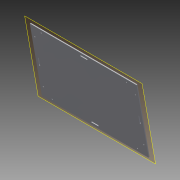
# Autodesk Inventor part: Panel_bottom
Saved by Autodesk Inventor 2013 (Build 170138000, 138)
## iProperties
Created: 2013-02-02
Part Number: Panel_bottom
Material: Aluminum 6061
Document SubType Name: Modeling
Designer: xylzlyx
Density: 1 g/cm^3
Author: xylzlyx
Autodesk Inventor part; units mm, degrees
ref_plane "YZ Plane" through (0, 0, 0) normal (1, 0, 0) x (0, 1, 0)
ref_plane "XZ Plane" through (0, 0, 0) normal (0, 1, 0) x (-1, 0, 0)
ref_plane "XY Plane" through (0, 0, 0) normal (0, 0, 1) x (1, 0, 0)
ref_plane "10DegOffset" through (-190.5, -127, 0) normal (0, -0.1736482, 0.9848078) x (1, 0, 0)
sketch "BottomDimensions" plane through (-190.5, -127, 0) normal (0, -0.1736482, 0.9848078) x (1, 0, 0)
  line L0 (380, 250.1412) -> (1, 250.1412) construction
  line L1 (0, 249.1564) -> (0, 0.9848) construction
  line L2 (381, 0.9848) -> (381, 249.1564) construction
  line L3 (1, 0) -> (380, 0) construction
  line L4 (0, 250.1412) -> (381, 250.1412)
  line L5 (381, 250.1412) -> (381, 0)
  line L6 (381, 0) -> (0, 0)
  line L7 (0, 0) -> (0, 250.1412)
  point P0 (190.5, 125.0706)
  constraints: 8 end point, 2 horizontal alignment, 2 parallel, 2 vertical alignment, 1 horizontal, 1 perpendicular
extrude "Panel" add sketch "BottomDimensions" along normal blind 3.175
fillet "CornerFillets" radius 1 4 edges at (-190.5, 119.0653, 44.9999) (190.5, 119.0653, 44.9999) (190.5, -127.2757, 1.5634) (-190.5, -127.2757, 1.5634)
sketch "ScrewHoleSketch" plane through (-190.5, -127.5513, 3.1268) normal (0, -0.1736482, 0.9848078) x (1, 0, 0)
  line L0 (9.525, 40.9987) -> (12.7, 40.9987) projected
  line L1 (12.7, 37.2014) -> (9.525, 37.2014) projected
  line L2 (12.7, 209.1425) -> (9.525, 209.1425) projected
  line L3 (9.525, 212.9398) -> (12.7, 212.9398) projected
  line L4 (39.9986, 240.6162) -> (39.9986, 237.4412) projected
  line L5 (36.2013, 237.4412) -> (36.2013, 240.6162) projected
  line L6 (188.6014, 237.4412) -> (188.6014, 240.6162) projected
  line L7 (192.3987, 240.6162) -> (192.3987, 237.4412) projected
  line L8 (344.7986, 240.6162) -> (344.7986, 237.4412) projected
  line L9 (341.0013, 237.4412) -> (341.0013, 240.6162) projected
  line L10 (371.475, 209.1425) -> (368.3, 209.1425) projected
  line L11 (368.3, 212.9398) -> (371.475, 212.9398) projected
  line L12 (368.3, 40.9986) -> (371.475, 40.9986) projected
  line L13 (371.475, 37.2013) -> (368.3, 37.2013) projected
  line L14 (341.0014, 9.525) -> (341.0014, 12.7) projected
  line L15 (344.7987, 12.7) -> (344.7987, 9.525) projected
  line L16 (192.3987, 12.7) -> (192.3987, 9.525) projected
  line L17 (188.6014, 9.525) -> (188.6014, 12.7) projected
  line L18 (36.2013, 9.525) -> (36.2013, 12.7) projected
  line L19 (39.9986, 12.7) -> (39.9986, 9.525) projected
  line L20 (9.525, 212.9398) -> (9.525, 209.1425) construction
  line L21 (39.9986, 240.6162) -> (36.2013, 240.6162) construction
  line L22 (344.7986, 240.6162) -> (341.0013, 240.6162) construction
  line L23 (371.475, 209.1425) -> (371.475, 212.9398) construction
  line L24 (368.3, 40.9986) -> (368.3, 37.2013) construction
  line L25 (344.7987, 12.7) -> (341.0014, 12.7) construction
  line L26 (36.2013, 9.525) -> (39.9986, 9.525) construction
  line L27 (12.7, 37.2014) -> (12.7, 40.9987) construction
  point P0 (190.5, 125.0706)
  point P1 (11.1125, 211.0412)
  point P2 (38.1, 239.0287)
  point P3 (342.9, 239.0287)
  point P4 (369.8875, 211.0412)
  point P5 (369.8875, 39.1)
  point P6 (342.9, 11.1125)
  point P7 (36.2013, 239.0287)
  point P8 (9.525, 211.0412)
  point P9 (38.1, 240.6162)
  point P10 (11.1125, 212.9398)
  point P11 (344.7986, 239.0287)
  point P12 (342.9, 240.6162)
  point P13 (369.8875, 212.9398)
  point P14 (371.475, 211.0412)
  point P15 (368.3, 39.1)
  point P16 (341.0014, 11.1125)
  point P17 (369.8875, 40.9986)
  point P18 (342.9, 12.7)
  point P19 (11.1125, 39.1)
  point P20 (38.1, 11.1125)
  point P21 (38.1, 9.525)
  point P22 (11.1125, 37.2014)
  point P23 (12.7, 39.1)
  point P24 (36.2013, 11.1125)
  constraints: 16 end point, 16 midpoint, 8 horizontal alignment, 8 vertical alignment, 2 parallel
hole "ScrewHoles" at (-179.3875, 80.2836, 39.7737) at (-152.4, 107.846, 44.6337) at (152.4, 107.846, 44.6337) at (179.3875, 80.2836, 39.7737) at (179.3875, -89.0453, 9.9164) at (152.4, -116.6077, 5.0564) at (-179.3875, -89.0453, 9.9164) at (-152.4, -116.6077, 5.0564) direction (0, 0.1736482, -0.9848078) diameter 3.7973 end through all
sketch "TabSlotSketch" plane through (-190.5, -127.5513, 3.1268) normal (0, -0.1736482, 0.9848078) x (1, 0, 0)
  circle A0 centre (38.1, 11.1125) radius 1.8986 projected
  circle A1 centre (342.9, 11.1125) radius 1.8986 projected
  circle A2 centre (369.8875, 211.0412) radius 1.8986 projected
  circle A3 centre (38.1, 239.0287) radius 1.8986 projected
  circle A4 centre (342.9, 239.0287) radius 1.8986 projected
  circle A5 centre (369.8875, 39.1) radius 1.8986 projected
  line L0 (12.7, 208.6425) -> (12.7, 41.4986) construction
  line L1 (9.525, 41.4986) -> (9.525, 208.6425) construction
  line L2 (9.525, 213.4398) -> (9.525, 236.4412) construction
  line L3 (12.7, 236.4412) -> (12.7, 213.4398) construction
  line L4 (35.7013, 237.4412) -> (1, 237.4412) construction
  line L5 (1, 240.6162) -> (35.7013, 240.6162) construction
  line L6 (9.525, 13.7) -> (9.525, 36.7013) construction
  line L7 (12.7, 36.7013) -> (12.7, 13.7) construction
  line L8 (1, 12.7) -> (35.7013, 12.7) construction
  line L9 (1, 9.525) -> (35.7013, 9.525) construction
  line L10 (345.2987, 9.525) -> (380, 9.525) construction
  line L11 (345.2987, 12.7) -> (380, 12.7) construction
  line L12 (368.3, 13.7) -> (368.3, 36.7013) construction
  line L13 (371.475, 36.7013) -> (371.475, 13.7) construction
  line L14 (371.475, 208.6425) -> (371.475, 41.4986) construction
  line L15 (368.3, 41.4986) -> (368.3, 208.6425) construction
  line L16 (368.3, 213.4398) -> (368.3, 236.4412) construction
  line L17 (371.475, 236.4412) -> (371.475, 213.4398) construction
  line L18 (380, 237.4412) -> (345.2986, 237.4412) construction
  line L19 (345.2986, 240.6162) -> (380, 240.6162) construction
  line L20 (340.5013, 237.4412) -> (40.4986, 237.4412) construction
  line L21 (40.4986, 240.6162) -> (340.5013, 240.6162) construction
  line L22 (40.4986, 9.525) -> (340.5014, 9.525) construction
  line L23 (40.4986, 12.7) -> (340.5014, 12.7) construction
  line L24 (13.0175, 138.4056) -> (9.2075, 138.4056)
  line L25 (9.2075, 138.4056) -> (9.2075, 111.7356)
  line L26 (9.2075, 111.7356) -> (13.0175, 111.7356)
  line L27 (13.0175, 111.7356) -> (13.0175, 138.4056)
  line L28 (371.7925, 111.7356) -> (367.9825, 111.7356)
  line L29 (367.9825, 111.7356) -> (367.9825, 138.4056)
  line L30 (367.9825, 138.4056) -> (371.7925, 138.4056)
  line L31 (371.7925, 138.4056) -> (371.7925, 111.7356)
  line L32 (9.525, 236.4412) -> (12.7, 236.4412) construction
  line L33 (9.525, 13.7) -> (12.7, 13.7) construction
  line L34 (11.1125, 13.7) -> (11.1125, 236.4412) construction
  line L35 (9.2075, 125.0706) -> (13.0175, 125.0706) construction
  line L36 (11.1125, 138.4056) -> (11.1125, 111.7356) construction
  line L37 (369.8875, 211.0412) -> (369.8875, 39.1) construction
  line L38 (177.165, 240.9337) -> (203.835, 240.9337)
  line L39 (203.835, 240.9337) -> (203.835, 237.1237)
  line L40 (203.835, 237.1237) -> (177.165, 237.1237)
  line L41 (177.165, 237.1237) -> (177.165, 240.9337)
  line L42 (177.165, 13.0175) -> (203.835, 13.0175)
  line L43 (203.835, 13.0175) -> (203.835, 9.2075)
  line L44 (203.835, 9.2075) -> (177.165, 9.2075)
  line L45 (177.165, 9.2075) -> (177.165, 13.0175)
  line L46 (38.1, 239.0287) -> (342.9, 239.0287) construction
  line L47 (38.1, 11.1125) -> (342.9, 11.1125) construction
  point P0 (190.5, 125.0706)
  point P1 (11.1125, 125.0706)
  point P2 (369.8875, 125.0706)
  point P3 (369.8875, 138.4056)
  point P4 (371.7925, 125.0706)
  point P5 (369.8875, 125.0706)
  point P6 (190.5, 239.0287)
  point P7 (190.5, 11.1125)
  point P8 (203.835, 239.0287)
  point P9 (203.835, 11.1125)
  point P10 (190.5, 240.9337)
  point P11 (190.5, 13.0175)
  point P12 (190.5, 239.0287)
  point P13 (190.5, 11.1125)
  dimension "d10" = 26.67
  dimension "d12" = 3.81
  dimension "d13" = 26.67
  dimension "d14" = 3.81
  dimension "d15" = 26.67
  dimension "d16" = 3.81
  dimension "d17" = 26.67
  dimension "d18" = 3.81
  constraints: 48 end point, 16 midpoint, 16 parallel, 4 horizontal, 4 perpendicular, 3 coincident, 3 horizontal alignment, 3 vertical alignment
  measures "d10" distance of L26.end L24.start
  measures "d12" distance of L25.end L26.end
  measures "d13" distance of L30.end L28.start
  measures "d14" distance of L29.end L30.end
  measures "d15" distance of L38.start L38.end
  measures "d16" distance of L38.end L39.end
  measures "d17" distance of L42.start L42.end
  measures "d18" distance of L42.end L43.end
extrude "TabSlotExtrusion" cut sketch "TabSlotSketch" against normal blind 3.175 contours L27 L26 L25 L24 | L28 L29 L30 L31 | L38 L39 L40 L41 | L42 L43 L44 L45
fillet "TabSlotFillets" radius 0.5 16 edges at (-177.4825, 9.0272, 25.5973) (-181.2925, 9.0272, 25.5973) (-177.4825, -17.2376, 20.9661) (-181.2925, -17.2376, 20.9661) (13.335, 109.9977, 43.4011) (13.335, 106.2456, 42.7395) (-13.335, 106.2456, 42.7395) (-13.335, 109.9977, 43.4011) (181.2925, 9.0272, 25.5973) (177.4825, 9.0272, 25.5973) (177.4825, -17.2376, 20.9661) (181.2925, -17.2376, 20.9661) (13.335, -114.4559, 3.8238) (-13.335, -114.4559, 3.8238) (-13.335, -118.208, 3.1622) (13.335, -118.208, 3.1622)
equation "\"d3\" = ScrewHoleD"
equation "\"d10\" = SlotLength"
equation "\"d12\" = SlotWidth"
equation "\"d13\" = SlotLength"
equation "\"d14\" = SlotWidth"
equation "\"d15\" = SlotLength"
equation "\"d16\" = SlotWidth"
equation "\"d17\" = SlotLength"
equation "\"d18\" = SlotWidth"
equation "\"d21\" = SlotFilletRad"
equation "\"ScrewHoleD\" = 3.7973"
equation "\"SlotLength\" = 26.67"
equation "\"SlotWidth\" = 3.81"
equation "\"SlotFilletRad\" = 0.5"
body "Solid1"
